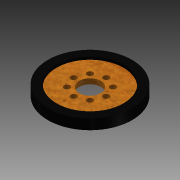
# Autodesk Inventor part: EncoderWheel
Saved by Autodesk Inventor 2014 SP1 (Build 180222100, 222)
## iProperties
Created: 2015-03-21
Part Number: EncoderWheel
Material: Rubber, Silicone
Document SubType Name: Modeling
Designer: david
Density: 1.25 g/cm^3
Appearance: Rubber - Black - Version 1.1
Mass: 8.91451 g
Surface Area: 50.4501 cm^2
Volume: 7.13161 cm^3
EncoderWheel_InnerDiameter: 39,000 mm
EncoderWheel_Tyre_Width: 6,000 mm
EncoderWheel_Tyre_SideWidth: 1,500 mm
EncoderWheel_Tyre_Diameter: 49,000 mm
EncoderWheel_FasteningHole_Diameter: 3,500 mm
EncoderWheel_FasteningHole_DistanceToCenter: 9,500 mm
Author: david
Autodesk Inventor part; units mm, degrees
ref_plane "YZ Plane" through (0, 0, 0) normal (1, 0, 0) x (0, 1, 0)
ref_plane "XZ Plane" through (0, 0, 0) normal (0, 1, 0) x (-1, 0, 0)
ref_plane "XY Plane" through (0, 0, 0) normal (0, 0, 1) x (1, 0, 0)
sketch "WheelSketch" plane through (0, 0, 0) normal (0, 1, 0) x (-1, 0, 0)
  circle A0 centre (0, 0) radius 24.5
  dimension "EncoderWheel_Tyre_Diameter" = 49
  constraints: 1 centre point, 1 coincident
  measures "EncoderWheel_Tyre_Diameter" diameter of A0
extrude "Wheel" add sketch "WheelSketch" along normal blind 6
sketch "Sketch2" plane through (0, 6, 0) normal (0, 1, 0) x (1, 0, 0)
  circle A0 centre (0, 0) radius 24.5 projected
  circle A1 centre (0, 0) radius 19.5
  dimension "EncoderWheel_Tyre_Thickness" = 5
  constraints: 1 centre point, 1 coincident
  measures "EncoderWheel_Tyre_Thickness" radial gap between concentric circles of A0 A1
extrude "Extrusion2" cut sketch "Sketch2" against normal blind 1.5 contours A1
sketch "Sketch3" plane through (0, 0, 0) normal (0, -1, 0) x (1, 0, 0)
  circle A0 centre (0, 0) radius 24.5 projected
  circle A1 centre (0, 0) radius 19.5
  dimension "d7" = 5
  constraints: 1 centre point, 1 coincident
  measures "d7" radial gap between concentric circles of A0 A1
extrude "Extrusion3" cut sketch "Sketch3" against normal blind 1.5 contours A1
sketch "InnerHoleSketch" plane through (0, 1.5, 0) normal (0, -1, 0) x (1, 0, 0)
  circle A0 centre (0, 0) radius 19.5 projected
  circle A1 centre (0, 0) radius 6.25
  dimension "EncoderWheel_InnerHole_Diameter" = 12.5
  constraints: 1 centre point, 1 coincident
  measures "EncoderWheel_InnerHole_Diameter" diameter of A1
extrude "InnerHole" cut sketch "InnerHoleSketch" against normal up to next contours A1
sketch "FasteningHoleSketch" plane through (0, 4.5, 0) normal (0, 1, 0) x (1, 0, 0)
  circle A0 centre (0, 0) radius 6.25 projected
  circle A1 centre (0, 0) radius 19.5 projected
  circle A2 centre (0, 9.5) radius 1.75
  line L0 (0, 0) -> (0, 29.2255) construction
  circle A3 centre (-6.7175, 6.7175) radius 1.75
  circle A4 centre (-9.5, 0) radius 1.75
  circle A5 centre (-6.7175, -6.7175) radius 1.75
  circle A6 centre (0, -9.5) radius 1.75
  circle A7 centre (6.7175, -6.7175) radius 1.75
  circle A8 centre (9.5, 0) radius 1.75
  circle A9 centre (6.7175, 6.7175) radius 1.75
  dimension "EncoderWheel_FasteningHole_Diameter" = 3.5
  dimension "EncoderWheel_FasteningHole_DistanceToCenter" = 9.5
  dimension "d17" = 360
  constraints: 8 centre point, 2 end point, 1 point on line, 1 vertical, 17 other
  measures "EncoderWheel_FasteningHole_Diameter" diameter of A2
  measures "EncoderWheel_FasteningHole_DistanceToCenter" distance of A0.centre A2.centre
extrude "FasteningHole" cut sketch "FasteningHoleSketch" against normal up to next contours A2 | A3 | A4 | A5 | A6 | A7 | A8 | A9
equation "\"d7\" = EncoderWheel_Tyre_Thickness"
equation "\"EncoderWheel_InnerDiameter\" = EncoderWheel_Tyre_Diameter - 2 * EncoderWheel_Tyre_Thickness"
body "Solid1"
